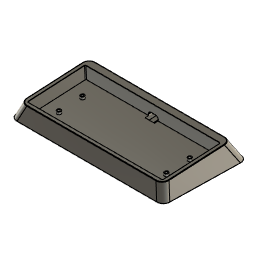
Bruce the Menhir (Autodesk Fusion 360 design; units mm, degrees)
Autodesk Fusion 360 part; units mm, degrees
sketch "Top Plane Sketch" plane through (0, 0, 0) normal (0, 0, 1) x (1, 0, 0)
  line L0 (-95.25, -40.4812) -> (95.25, -40.4812) construction
  line L1 (95.25, -40.4812) -> (95.25, 40.4812) construction
  line L2 (95.25, 40.4812) -> (-95.25, 40.4812) construction
  line L3 (-95.25, 40.4812) -> (-95.25, -40.4812) construction
  line L4 (-95.75, -40.9812) -> (95.75, -40.9812)
  line L5 (95.75, -40.9812) -> (95.75, 40.9812)
  line L6 (95.75, 40.9813) -> (-95.75, 40.9813)
  line L7 (-95.75, 40.9813) -> (-95.75, -40.9812)
  line L8 (-100.75, -45.9812) -> (100.75, -45.9812)
  line L9 (100.75, -45.9812) -> (100.75, 50.9812)
  line L10 (100.75, 50.9813) -> (-100.75, 50.9813)
  line L11 (-100.75, 50.9813) -> (-100.75, -45.9812)
  line L12 (-95.25, 40.4812) -> (95.25, -40.4812) construction
  line L13 (95.25, 40.4812) -> (-95.25, -40.4812) construction
  circle A0 centre (0, 0) radius 1.8249 construction
  dimension "d1" = 190.5
  dimension "d2" = 80.9625
  dimension "d3" = 0.5
  dimension "d9" = 10
  dimension "d10" = 5
  dimension "d11" = 5
  dimension "d12" = 5
  constraint horizontal L0
  constraint vertical L1
  constraint horizontal L2
  constraint vertical L3
  constraint midpoint L12 A0.centre
  measures "d1" distance of L0.start L0.end
  measures "d2" distance of L0.start L2.end
  measures "d9" distance of L6 L10
  measures "d10" distance of L7 L11
  measures "d11" distance of L5 L9
  measures "d12" distance of L4 L8
ref_plane "WorkPlane1" through (0, 0, -50) normal (0, 0, 1) x (1, 0, 0)
sketch "Base Plane Sketch" plane through (0, 0, -50) normal (0, 0, 1) x (1, 0, 0)
  line L0 (95.25, -40.4813) -> (-95.25, -40.4813) construction
  line L1 (-95.25, -40.4813) -> (-95.25, 40.4812) construction
  line L2 (-95.25, 40.4812) -> (95.25, 40.4812) construction
  line L3 (95.25, 40.4812) -> (95.25, -40.4813) construction
  line L4 (95.25, -40.4813) -> (-95.25, 40.4813) construction
  line L5 (-95.25, -40.4813) -> (95.25, 40.4812) construction
  circle A0 centre (0, 0) radius 6.9017 construction
  line L6 (95.75, -40.9813) -> (-95.75, -40.9813) construction
  line L7 (-95.75, -40.9813) -> (-95.75, 40.9812) construction
  line L8 (-95.75, 40.9812) -> (95.75, 40.9812) construction
  line L9 (95.75, 40.9812) -> (95.75, -40.9812) construction
  line L10 (-100.75, 50.9812) -> (100.75, 50.9812) construction
  line L11 (100.75, 50.9812) -> (100.75, -45.9812) construction
  line L12 (100.75, -45.9813) -> (-100.75, -45.9813) construction
  line L13 (-100.75, -45.9813) -> (-100.75, 50.9812) construction
  line L14 (-120.75, 74.9813) -> (120.75, 74.9813)
  line L15 (120.75, 74.9813) -> (120.75, -65.9813)
  line L16 (120.75, -65.9813) -> (-120.75, -65.9812)
  line L17 (-120.75, -65.9812) -> (-120.75, 74.9812)
  dimension "d14" = 190.5
  dimension "d15" = 80.9625
  dimension "d16" = -0.5
  dimension "d17" = 10
  dimension "d18" = 5
  dimension "d19" = 5
  dimension "d20" = 5
  dimension "d21" = 20
  dimension "d22" = 20
  dimension "d23" = 20
  dimension "d24" = 24
  constraint horizontal L0
  constraint perpendicular L0 L1
  constraint parallel L0 L2
  constraint parallel L1 L3
  constraint coincident L4 A0.centre
  constraint coincident L5 A0.centre
  constraint coincident A0.centre origin
  constraint horizontal L10
  constraint vertical L11
  constraint horizontal L12
  constraint vertical L13
  constraint horizontal L14
  constraint vertical L15
  constraint horizontal L16
  constraint vertical L17
  measures "d14" distance of L1.end L2.end
  measures "d15" distance of L0.end L1.end
  measures "d17" distance of L8 L10
  measures "d18" distance of L7 L13
  measures "d19" distance of L9 L11
  measures "d20" distance of L6 L12
  measures "d21" distance of L12 L16
  measures "d22" distance of L11 L15
  measures "d23" distance of L13 L17
  measures "d24" distance of L10 L14
loft "Loft1" add profiles "Top Plane Sketch", "Base Plane Sketch" section 1 section 2
sketch "Angle Cut Line" plane through (0, -39.639, 15.8556) normal (0, -0.928477, 0.371391) x (1, 0, 0)
  line L0 (100.75, -17.077) -> (-100.75, -17.077)
  line L1 (-100.75, -17.077) -> (-120.75, -70.9287)
  line L2 (-120.75, -70.9287) -> (120.75, -70.9287)
  line L3 (120.75, -70.9287) -> (100.75, -17.077)
  line L4 (-108.5492, -38.077) -> (108.5492, -38.077)
  dimension "d37" = 21
  constraint coincident L1 L4.start
  constraint coincident L3 L4.end
  constraint parallel L2 L4
  measures "d37" distance of L0 L4
ref_plane "WorkPlane2" through (0, -53.7805, -19.498) normal (0, 0.052336, 0.99863) x (1, 0, 0)
extrude "Extrude1" cut 1 faces at (-40.25, 27.9937, -50) along direction (0, 0, -1) up to surface end surface through (0, -53.7805, -19.498) normal (0, 0.052336, 0.99863) offset 0
fillet "Fillet1" radius 10 4 edges at (-105.8766, 57.1332, -12.8166) (-104.6496, -49.8809, -9.749) (104.6496, -49.8809, -9.749) (105.8766, 57.1332, -12.8166)
extrude "Extrude2" cut sketch "Top Plane Sketch" against normal blind 18.06 contours L4 L5 L6 L7
fillet "Fillet2" radius 1 4 edges at (-95.75, 40.9813, -9.03) (95.75, 40.9813, -9.03) (95.75, -40.9812, -9.03) (-95.75, -40.9812, -9.03)
chamfer "Chamfer1" distance 0.5 angle 45 8 edges at (0, -45.9812, 0) (98.1037, -43.335, 0) (100.75, 2.4876, 0) (98.1846, 48.3392, 0) (0, 50.9813, 0) (-98.1846, 48.3392, 0) (-100.75, 2.4876, 0) (-98.1037, -43.335, 0)
chamfer "Chamfer3" distance 0.25 angle 45 8 edges at (0, 40.9813, 0) (95.4571, 40.6884, 0) (95.75, 0, 0) (95.4571, -40.6884, 0) (0, -40.9812, 0) (-95.4571, -40.6884, 0) (-95.75, 0, 0) (-95.4571, 40.6884, 0)
chamfer "Chamfer4" distance 0.5 angle 45 8 edges at (-109.7715, 4.5245, -22.5536) (-105.9572, -51.1885, -19.6338) (0, -53.7805, -19.498) (105.9572, -51.1885, -19.6338) (109.7715, 4.5245, -22.5536) (108.3811, 60.5749, -25.4911) (0, 63.2852, -25.6332) (-108.3811, 60.5749, -25.4911)
sketch "Screw Post Sketch" plane through (0, 0, -18.06) normal (0, 0, 1) x (1, 0, 0)
  arc A0 (-95.75, -39.9812) -> (-94.75, -40.9812) centre (-94.75, -39.9812) ccw
  line L0 (-94.75, -40.9812) -> (94.75, -40.9812)
  arc A1 (94.75, -40.9813) -> (95.75, -39.9813) centre (94.75, -39.9813) ccw
  line L1 (95.75, -39.9813) -> (95.75, 39.9813)
  arc A2 (95.75, 39.9812) -> (94.75, 40.9813) centre (94.75, 39.9813) ccw
  line L2 (94.75, 40.9813) -> (-94.75, 40.9813)
  arc A3 (-94.75, 40.9813) -> (-95.75, 39.9813) centre (-94.75, 39.9813) ccw
  line L3 (-95.75, 39.9813) -> (-95.75, -39.9812)
  circle A4 centre (-76.2, 16.6688) radius 2.75
  circle A5 centre (76.2, 16.6687) radius 2.75
  circle A6 centre (76.2, -16.6687) radius 2.75
  circle A7 centre (-76.2, -16.6687) radius 2.75
  circle A8 centre (-76.2, 16.6688) radius 1.6
  circle A9 centre (-76.2, -16.6687) radius 1.6
  circle A10 centre (76.2, 16.6687) radius 1.6
  circle A11 centre (76.2, -16.6687) radius 1.6
  arc A12 (-95.75, -39.9812) -> (-94.75, -40.9812) centre (-94.75, -39.9812) ccw
  line L4 (-94.75, -40.9812) -> (94.75, -40.9812)
  arc A13 (94.75, -40.9813) -> (95.75, -39.9813) centre (94.75, -39.9813) ccw
  line L5 (95.75, -39.9813) -> (95.75, 39.9813)
  arc A14 (95.75, 39.9812) -> (94.75, 40.9813) centre (94.75, 39.9813) ccw
  line L6 (94.75, 40.9813) -> (-94.75, 40.9813)
  arc A15 (-94.75, 40.9813) -> (-95.75, 39.9813) centre (-94.75, 39.9813) ccw
  line L7 (-95.75, 39.9813) -> (-95.75, -39.9812)
  arc A16 (-95.75, -39.9812) -> (-94.75, -40.9812) centre (-94.75, -39.9812) ccw
  line L8 (-94.75, -40.9812) -> (94.75, -40.9812)
  arc A17 (94.75, -40.9813) -> (95.75, -39.9813) centre (94.75, -39.9813) ccw
  line L9 (95.75, -39.9813) -> (95.75, 39.9813)
  arc A18 (95.75, 39.9812) -> (94.75, 40.9813) centre (94.75, 39.9813) ccw
  line L10 (94.75, 40.9813) -> (-94.75, 40.9813)
  arc A19 (-94.75, 40.9813) -> (-95.75, 39.9813) centre (-94.75, 39.9813) ccw
  line L11 (-95.75, 39.9813) -> (-95.75, -39.9812)
  line L12 (-95.25, 39.9813) -> (-95.25, -39.9812) construction
  arc A20 (-95.25, -39.9812) -> (-94.75, -40.4812) centre (-94.75, -39.9812) ccw construction
  line L13 (-94.75, -40.4812) -> (94.75, -40.4812) construction
  arc A21 (94.75, -40.4813) -> (95.25, -39.9813) centre (94.75, -39.9813) ccw construction
  line L14 (95.25, -39.9813) -> (95.25, 39.9813) construction
  arc A22 (95.25, 39.9812) -> (94.75, 40.4812) centre (94.75, 39.9813) ccw construction
  line L15 (94.75, 40.4812) -> (-94.75, 40.4813) construction
  arc A23 (-94.75, 40.4813) -> (-95.25, 39.9813) centre (-94.75, 39.9813) ccw construction
  dimension "d41" = 5.5
  dimension "d52" = 3.2
  dimension "d53" = 3.2
  dimension "d54" = 3.2
  dimension "d55" = 3.2
  dimension "d68" = -0.5
  dimension "d69" = 23.8125
  dimension "d70" = 19.05
  dimension "d71" = 23.8125
  dimension "d72" = 19.05
  dimension "d73" = 19.05
  dimension "d74" = 23.8125
  dimension "d75" = 23.8125
  dimension "d76" = 19.05
  constraint equal A4 A5
  constraint equal A4 A7
  constraint equal A4 A6
  constraint concentric A4 A8
  constraint concentric A7 A9
  constraint concentric A5 A10
  constraint concentric A6 A11
  measures "d41" diameter of A4
  measures "d52" diameter of A8
  measures "d53" diameter of A9
  measures "d54" diameter of A10
  measures "d55" diameter of A11
  measures "d69" distance of A4.centre L15
  measures "d70" distance of A4.centre L12
  measures "d71" distance of A5.centre L15
  measures "d72" distance of A5.centre L14
  measures "d73" distance of A6.centre L14
  measures "d74" distance of A6.centre L13
  measures "d75" distance of A7.centre L13
  measures "d76" distance of A7.centre L12
extrude "Extrude3" add sketch "Screw Post Sketch" along normal blind 3.46 contours A4 | A5 | A6 | A7 | A8 | A9 | A10 | A11
extrude "Extrude4" cut sketch "Screw Post Sketch" along normal blind 3.46 and the other way blind 0.54 contours A8 | A9 | A10 | A11
sketch "USB C Hole" plane through (0, 40.9813, 0) normal (0, -1, 0) x (1, 0, 0)
  line L0 (94.75, -0.25) -> (-94.75, -0.25)
  line L1 (-94.75, -0.25) -> (-94.75, -18.06)
  line L2 (-94.75, -18.06) -> (94.75, -18.06)
  line L3 (94.75, -18.06) -> (94.75, -0.25)
  line L4 (0, -18.06) -> (0, -16.23) construction
  line L5 (6.975, -12.15) -> (-6.975, -12.15)
  line L6 (-6.975, -12.15) -> (-6.975, -20.31)
  line L7 (-6.975, -20.31) -> (6.975, -20.31)
  line L8 (6.975, -20.31) -> (6.975, -12.15)
  line L9 (6.975, -12.15) -> (-6.975, -20.31) construction
  line L10 (-6.975, -12.15) -> (6.975, -20.31) construction
  point P0 (0, -16.23)
  dimension "d60" = 1.83
  dimension "d61" = 13.95
  dimension "d62" = 8.16
  constraint midpoint L2 L4.start
  constraint perpendicular L2 L4
  constraint horizontal L5
  constraint perpendicular L5 L6
  constraint parallel L5 L7
  constraint parallel L6 L8
  constraint coincident L9 P0
  constraint coincident L10 P0
  constraint coincident P0 L4.end
  measures "d60" distance of L4.start P0
  measures "d61" distance of L6.end L7.end
  measures "d62" distance of L5.end L6.end
extrude "Extrude5" cut sketch "USB C Hole" along normal blind -25 and the other way blind -5 contours L2 L6 L7 L8 | L2 L5 L6 L8
fillet "Fillet3" radius 3.8 4 edges at (6.975, 48.3557, -20.31) (6.975, 48.8973, -12.15) (-6.975, 48.3557, -20.31) (-6.975, 48.8973, -12.15)
chamfer "Chamfer5" distance 0.25 angle 45 8 edges at (0, 56.8133, -12.15) (-5.862, 57.3475, -13.263) (-6.975, 58.7717, -16.23) (-5.862, 60.1958, -19.197) (0, 60.7301, -20.31) (5.862, 60.1958, -19.197) (6.975, 58.7717, -16.23) (5.862, 57.3475, -13.263)
move_body "Move2" bodies 1 to x (1, 0, 0) y (0, 0.99863, 0.052336) z (0, -0.052336, 0.99863) at (0, -1.0948, 2.7618)
equation "d1 = 19.05 mm * 10"
equation "d2 = 19.05 mm * 4.25"
equation "d14 = 19.05 mm * 10"
equation "d15 = 19.05 mm * 4.25"
equation "d17 = d9"
equation "d18 = d10"
equation "d19 = d11"
equation "d20 = d12"
equation "d21 = 10 mm * 2"
equation "d22 = d21"
equation "d23 = d21"
equation "d24 = 12 mm * 2"
equation "d25 = -3 deg"
equation "d53 = d52"
equation "d54 = d52"
equation "d55 = d52"
equation "d58 = 4 mm - 3.46 mm"
equation "d60 = ( 3.66 / 2 ) * 1 mm"
equation "d69 = 19.05 mm * 1.25"
equation "d71 = d69"
equation "d72 = d70"
equation "d73 = d70"
equation "d74 = d69"
equation "d75 = d69"
equation "d76 = d70"
equation "d79 = -d25"
named bodies: "Bruce the Menhir"
